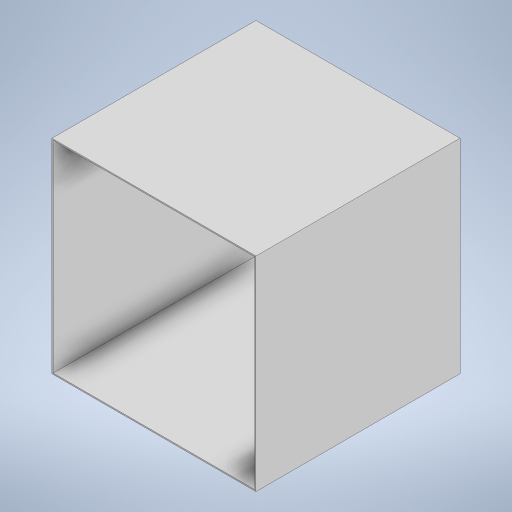
# Autodesk Inventor part: BOX
Saved by Autodesk Inventor 2024 (Build 280153000, 153)
## iProperties
Created: 2023-05-22
Part Number: BOX
Material: Genérico
Document SubType Name: Modeling
Designer: sebas
Density: 1 g/cm^3
Appearance: Valor por defecto
Author: sebas
Autodesk Inventor part; units mm, degrees
ref_plane "YZ Plane" through (0, 0, 0) normal (1, 0, 0) x (0, 1, 0)
ref_plane "XZ Plane" through (0, 0, 0) normal (0, 1, 0) x (-1, 0, 0)
ref_plane "XY Plane" through (0, 0, 0) normal (0, 0, 1) x (1, 0, 0)
sketch "Boceto1" plane through (0, 0, 0) normal (0, 0, 1) x (1, 0, 0)
  line L0 (-200, -200) -> (200, -200)
  line L1 (200, -200) -> (200, 200)
  line L2 (200, 200) -> (-200, 200)
  line L3 (-200, 200) -> (-200, -200)
  line L4 (-200, -200) -> (200, 200) construction
  line L5 (200, -200) -> (-200, 200) construction
  line L6 (-197.5, -197.5) -> (197.5, -197.5)
  line L7 (197.5, -197.5) -> (197.5, 197.5)
  line L8 (197.5, 197.5) -> (-197.5, 197.5)
  line L9 (-197.5, 197.5) -> (-197.5, -197.5)
  line L10 (-197.5, -197.5) -> (197.5, 197.5) construction
  line L11 (197.5, -197.5) -> (-197.5, 197.5) construction
  point P0 (0, 0)
  dimension "d0" = 400
  dimension "d1" = 400
  dimension "d2" = 395
  dimension "d3" = 395
  constraints: 24 end point, 4 midpoint, 4 parallel, 2 horizontal, 2 perpendicular
  measures "d0" distance of L2.end L1.end
  measures "d1" distance of L1.end L0.end
  measures "d2" distance of L8.end L7.end
  measures "d3" distance of L7.end L6.end
extrude "Extrusión1" add sketch "Boceto1" along normal blind 5 contours L9 L8 L7 L6
extrude "Extrusión2" add sketch "Boceto1" along normal blind 400
